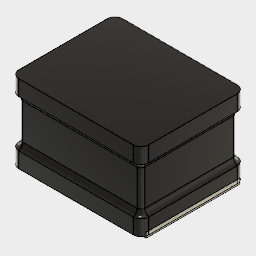
ind2520 (Autodesk Fusion 360 design; units mm, degrees)
Autodesk Fusion 360 part; units mm, degrees
note: some values were not read from the file. Chosen so that the rebuilt part matches the saved one: which face or edge a step refers to. Set by a fixed rule: which sketch regions a step uses.
ref_plane "WorkPlane3" through (0, 0, 0.03) normal (0, 0, 1) x (1, 0, 0)
sketch "Sketch1" plane through (0, 0, 0.03) normal (0, 0, 1) x (1, 0, 0)
  line L0 (1.1, 1) -> (-1.1, 1)
  line L1 (-1.25, 0.85) -> (-1.25, -0.85)
  line L2 (-1.1, -1) -> (1.1, -1)
  line L3 (1.25, -0.85) -> (1.25, 0.85)
  line L4 (1.25, 1) -> (-1.25, -1) construction
  line L5 (-1.25, 1) -> (1.25, -1) construction
  line L6 (0, 1) -> (0, -1) construction
  arc A0 (-1.25, -0.85) -> (-1.1, -1) centre (-1.1, -0.85) ccw
  arc A1 (1.1, -1) -> (1.25, -0.85) centre (1.1, -0.85) ccw
  arc A2 (1.25, 0.85) -> (1.1, 1) centre (1.1, 0.85) ccw
  arc A3 (-1.1, 1) -> (-1.25, 0.85) centre (-1.1, 0.85) ccw
  point P0 (1.05, 0)
  dimension "d10" = 2.5
  dimension "d11" = 2
  dimension "d30" = 0.15
  measures "d10" distance of L4.end L5.end
  measures "d11" distance of L5.start L4.end
  measures "d30" radius of A0
ref_plane "WorkPlane2" through (1.1, 0, 0) normal (1, 0, 0) x (0, 1, 0)
sketch "Sketch2" plane through (1.1, 0, 0) normal (1, 0, 0) x (0, 1, 0)
  line L0 (0, 0.03) -> (0, 1.53)
  line L1 (0, 1.53) -> (-1, 1.53)
  line L2 (-1, 1.53) -> (-1, 1.23)
  arc A0 (-0.925, 1.1239) -> (-1, 1.23) centre (-1.0375, 1.1239) ccw
  line L3 (-0.925, 1.1239) -> (-0.925, 0.4361)
  line L4 (-1, 0.03) -> (-1, 0.33)
  arc A1 (-1, 0.33) -> (-0.925, 0.4361) centre (-1.0375, 0.4361) ccw
  line L5 (-0.85, 1.53) -> (-0.85, 0.03)
  line L6 (0, 0.03) -> (-1, 0.03)
  point P0 (-0.85, 0.03)
  dimension "d22" = 0.075
  dimension "d23" = 0.3
  dimension "d24" = 0.3
  dimension "d26" = 0.1125
  dimension "d44" = 1.5
  dimension "d45" = 1
  measures "d22" distance of L3 L4.start
  measures "d23" distance of L1.end L2.end
  measures "d24" distance of L4.start L4.end
  measures "d26" radius of A1
  measures "d44" distance of L1 L6
  measures "d45" distance of L0 L2
sweep "Sweep1" add profiles "Sketch2" path "Sketch1" along A2 L0 A3 L1 A0 L2 A1 L3 section 1 contours L1 L2 A0 L3 L4 A1 L5 L6 makes body 1
sketch "Sketch3" plane through (0, 0, 1.53) normal (0, 0, 1) x (-1, 0, 0)
  line L0 (-1.1, 0.85) -> (1.1, 0.85)
  line L1 (1.1, 0.85) -> (1.1, -0.85)
  line L2 (1.1, -0.85) -> (-1.1, -0.85)
  line L3 (-1.1, -0.85) -> (-1.1, 0.85)
  arc A0 (-1.1, 1) -> (-1.25, 0.85) centre (-1.1, 0.85) ccw
  line L4 (-1.25, 0.85) -> (-1.25, -0.85)
  arc A1 (-1.25, -0.85) -> (-1.1, -1) centre (-1.1, -0.85) ccw
  line L5 (-1.1, -1) -> (1.1, -1)
  arc A2 (1.1, -1) -> (1.25, -0.85) centre (1.1, -0.85) ccw
  line L6 (1.25, -0.85) -> (1.25, 0.85)
  arc A3 (1.25, 0.85) -> (1.1, 1) centre (1.1, 0.85) ccw
  line L7 (1.1, 1) -> (-1.1, 1)
extrude "Extrude4" add sketch "Sketch3" against normal blind 1.5 contours L0 L1 L2 L3 bodies 1
sketch "Sketch4" plane through (0, 0, 0) normal (0, 0, 1) x (1, 0, 0)
  line L0 (-0.63, 0.9) -> (-1.25, 0.9)
  line L1 (-1.25, 0.9) -> (-1.25, -0.9)
  line L2 (-1.25, -0.9) -> (-0.63, -0.9)
  line L3 (-0.63, -0.9) -> (-0.63, 0.9)
  line L4 (-0.63, 0.9) -> (-1.25, -0.9) construction
  line L5 (-1.25, 0.9) -> (-0.63, -0.9) construction
  line L6 (0, 0) -> (0, 1.8014) construction
  line L7 (0.63, -0.9) -> (0.63, 0.9)
  line L8 (0.63, 0.9) -> (1.25, 0.9)
  line L9 (1.25, 0.9) -> (1.25, -0.9)
  line L10 (1.25, -0.9) -> (0.63, -0.9)
  point P0 (-0.94, 0)
  dimension "d48" = 1.8
  dimension "d50" = 0.63
  dimension "d51" = 1.25
  measures "d48" distance of L0 L2
  measures "d50" distance of L3 L6
  measures "d51" distance of L1 L6
extrude "Extrude5" add sketch "Sketch4" along normal blind 0.1 separate body makes body 2 at (-1.0433, 0.3, 0) makes body 3 at (1.0433, 0.3, 0)
equation "ind2520_package_length = 2.5 mm" comment "2.4 - 2.8"
equation "ind2520_package_width = 2 mm" comment "1.5 - 1.9"
equation "ind2520_package_height = 1.5 mm" comment "0.9 - 1.1"
equation "ind2520_above_board = 0.03 mm"
equation "ind2520_lead_thick = 0.1 mm" comment "0.1 - 0.22"
equation "ind2520_lead_width = ind2520_package_width - 0.2 mm" comment "0.75 - 1.05"
equation "ind2520_lead_extension = 0 mm" comment "0.3 - 0.6"
equation "d10 = ind2520_package_length"
equation "d11 = ind2520_package_width"
equation "d26 = d22 * 3 / 2"
equation "d33 = ind2520_package_length / 2 - d30"
equation "d44 = ind2520_package_height"
equation "d45 = ind2520_package_width / 2"
equation "d46 = ind2520_above_board"
equation "d47 = -ind2520_package_height"
equation "d48 = ind2520_lead_width"
equation "ind2520_lead_length = 0.62 mm"
equation "d50 = ind2520_package_length / 2 - ind2520_lead_length"
equation "d51 = ind2520_package_length / 2 + ind2520_lead_extension"
equation "d52 = ind2520_lead_thick"
